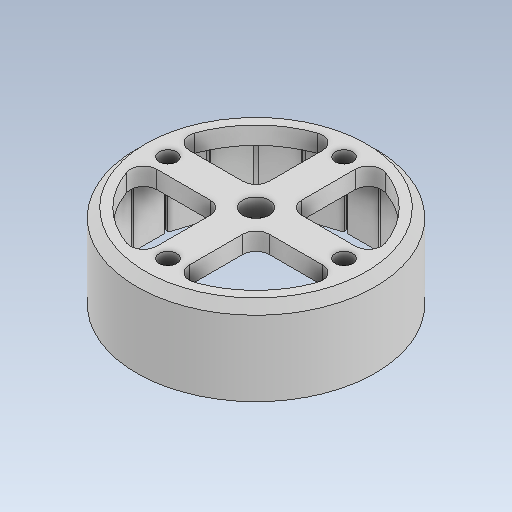
# Autodesk Inventor part: mot_27_1
Saved by Autodesk Inventor 2023 (Build 270158000, 158)
## iProperties
Created: 2020-12-02
Part Number: mot_27_1
Material: Generic
Document SubType Name: Modeling
Designer: Shuang Peng
Density: 1 g/cm^3
Appearance: Default
Author: Shuang Peng
Autodesk Inventor part; units mm, degrees
ref_plane "YZ Plane" through (0, 0, 0) normal (1, 0, 0) x (0, 1, 0)
ref_plane "XZ Plane" through (0, 0, 0) normal (0, 1, 0) x (-1, 0, 0)
ref_plane "XY Plane" through (0, 0, 0) normal (0, 0, 1) x (1, 0, 0)
sketch "Sketch1" plane through (0, 0, 0) normal (0, 1, 0) x (-1, 0, 0)
  circle A0 centre (0, 0) radius 13.55
  dimension "d0" = 27.1
  constraints: 1 centre point, 1 coincident
  measures "d0" diameter of A0
extrude "Extrusion1" add sketch "Sketch1" along normal blind 9.5
sketch "Sketch2" plane through (0, 9.5, 0) normal (0, 1, 0) x (1, 0, 0)
  circle A0 centre (0, 0) radius 13.55 projected
  line L0 (-1.85, -20) -> (1.85, -20)
  line L1 (1.85, -20) -> (1.85, 20)
  line L2 (1.85, 20) -> (-1.85, 20)
  line L3 (-1.85, 20) -> (-1.85, -20)
  line L4 (-1.85, -20) -> (1.85, 20) construction
  line L5 (1.85, -20) -> (-1.85, 20) construction
  line L6 (-20, -1.85) -> (-20, 1.85)
  line L7 (-20, 1.85) -> (20, 1.85)
  line L8 (20, 1.85) -> (20, -1.85)
  line L9 (20, -1.85) -> (-20, -1.85)
  line L10 (-20, -1.85) -> (20, 1.85) construction
  line L11 (-20, 1.85) -> (20, -1.85) construction
  circle A1 centre (0, 0) radius 11.5
  point P0 (1.85, -11.3502)
  point P1 (11.3502, -1.85)
  point P2 (1.85, -1.85)
  point P3 (11.3502, 1.85)
  point P4 (1.85, 11.3502)
  point P5 (1.85, 1.85)
  point P6 (-1.85, 11.3502)
  point P7 (-11.3502, 1.85)
  point P8 (-1.85, 1.85)
  point P9 (-11.3502, -1.85)
  point P10 (-1.85, -11.3502)
  point P11 (-1.85, -1.85)
  dimension "d3" = 3.7
  dimension "d4" = 40
  dimension "d5" = 3.7
  dimension "d6" = 40
  dimension "d7" = 23
  constraints: 24 end point, 4 midpoint, 4 parallel, 3 perpendicular, 1 centre point, 1 coincident, 1 horizontal
  measures "d3" distance of L0.start L0.end
  measures "d4" distance of L1.end L0.end
  measures "d5" distance of L6.start L6.end
  measures "d6" distance of L6.end L7.end
  measures "d7" diameter of A1
extrude "Extrusion2" cut sketch "Sketch2" against normal blind 9.5 contours L7 L1 A1 | A1 L1 L9 | L3 L7 A1 | A1 L9 L3
sketch "Sketch3" plane through (0, 0, 0) normal (0, -1, 0) x (1, 0, 0)
  line L0 (1.85, -11.3502) -> (1.85, -1.85) projected
  line L1 (1.85, -1.85) -> (11.3502, -1.85) projected
  arc A0 (1.85, -11.3502) -> (11.3502, -1.85) centre (0, 0) ccw projected
  line L2 (-11.3502, -1.85) -> (-1.85, -1.85) projected
  line L3 (-1.85, -1.85) -> (-1.85, -11.3502) projected
  arc A1 (-11.3502, -1.85) -> (-1.85, -11.3502) centre (0, 0) ccw projected
  line L4 (1.85, 1.85) -> (1.85, 11.3502) projected
  arc A2 (11.3502, 1.85) -> (1.85, 11.3502) centre (0, 0) ccw projected
  line L5 (11.3502, 1.85) -> (1.85, 1.85) projected
  arc A3 (-1.85, 11.3502) -> (-11.3502, 1.85) centre (0, 0) ccw projected
  line L6 (-1.85, 11.3502) -> (-1.85, 1.85) projected
  line L7 (-1.85, 1.85) -> (-11.3502, 1.85) projected
  circle A4 centre (0, 0) radius 13.55 projected
  circle A5 centre (0, 0) radius 12.7
  circle A6 centre (0, 0) radius 13.55 projected
  dimension "d10" = 0.85
  constraints: 1 centre point, 1 coincident
  measures "d10" radial gap between concentric circles of A6 A5
extrude "Extrusion3" cut sketch "Sketch3" against normal blind 7.5 contours A5
chamfer "Chamfer1" distance 1 angle 45 1 edges at (13.55, 9.5, 0)
sketch "Sketch4" plane through (0, 9.5, 0) normal (0, 1, 0) x (1, 0, 0)
  circle A0 centre (0, 0) radius 1.5
  dimension "d17" = 3
  constraints: 1 centre point, 1 coincident
  measures "d17" diameter of A0
extrude "Extrusion4" cut sketch "Sketch4" against normal blind 7.5
sketch "Sketch5" plane through (0, 7.5, 0) normal (0, -1, 0) x (1, 0, 0)
  circle A0 centre (0, 0) radius 1.5 projected
  circle A1 centre (0, 0) radius 12.7 projected
  line L0 (-11.3502, 1.85) -> (-1.85, 1.85) projected
  arc A2 (-1.85, 11.3502) -> (-11.3502, 1.85) centre (0, 0) ccw projected
  line L1 (-1.85, 1.85) -> (-1.85, 11.3502) projected
  line L2 (1.85, 1.85) -> (11.3502, 1.85) projected
  line L3 (1.85, 11.3502) -> (1.85, 1.85) projected
  arc A3 (11.3502, 1.85) -> (1.85, 11.3502) centre (0, 0) ccw projected
  arc A4 (-11.3502, -1.85) -> (-1.85, -11.3502) centre (0, 0) ccw projected
  line L4 (-1.85, -1.85) -> (-11.3502, -1.85) projected
  line L5 (-1.85, -11.3502) -> (-1.85, -1.85) projected
  line L6 (1.85, -1.85) -> (1.85, -11.3502) projected
  line L7 (11.3502, -1.85) -> (1.85, -1.85) projected
  arc A5 (1.85, -11.3502) -> (11.3502, -1.85) centre (0, 0) ccw projected
  circle A6 centre (0, 0) radius 12.7 projected
  line L8 (0, 0) -> (0, -12.5)
  line L9 (1.75, -12.85) -> (1.75, -12.15)
  line L10 (1.75, -12.15) -> (-1.75, -12.15)
  line L11 (-1.75, -12.15) -> (-1.75, -12.85)
  line L12 (-1.75, -12.85) -> (1.75, -12.85)
  line L13 (1.75, -12.85) -> (-1.75, -12.15) construction
  line L14 (1.75, -12.15) -> (-1.75, -12.85) construction
  dimension "d20" = 12.5
  dimension "d21" = 0.7
  dimension "d22" = 3.5
  constraints: 14 end point, 2 midpoint, 2 parallel, 2 perpendicular, 1 vertical
  measures "d20" distance of L8.start L8.end
  measures "d21" distance of L9.start L9.end
  measures "d22" distance of L10.end L9.end
extrude "Extrusion5" add sketch "Sketch5" along normal blind 7.5 contours L11 L10 L9 A1 | A1 L9 L12 L11 picked at (-0.7783, -12.3288)
pattern_circular "Circular Pattern1" count 20 over 360 about axis through (0, 0, 0) along (0, 1, 0) of "Extrusion5"
sketch "Sketch6" plane through (0, 9.5, 0) normal (0, 1, 0) x (1, 0, 0)
  line L0 (0, 0) -> (0, 10)
  circle A0 centre (0, 10) radius 1
  circle A1 centre (-10, 0) radius 1
  circle A2 centre (0, -10) radius 1
  circle A3 centre (10, 0) radius 1
  dimension "d28" = 10
  dimension "d29" = 2
  dimension "d32" = 360
  constraints: 4 centre point, 2 end point, 1 coincident, 1 vertical, 9 other
  measures "d28" distance of L0.start L0.end
  measures "d29" diameter of A0
extrude "Extrusion6" cut sketch "Sketch6" against normal blind 7.5
fillet "Fillet2" radius 1.5 12 edges at (1.85, 8.5, -1.85) (1.85, 8.5, 1.85) (-1.85, 8.5, -1.85) (-1.85, 8.5, 1.85) (-11.3502, 8.5, 1.85) (11.3502, 8.5, 1.85) (-11.3502, 8.5, -1.85) (11.3502, 8.5, -1.85) (-1.85, 8.5, -11.3502) (-1.85, 8.5, 11.3502) (1.85, 8.5, -11.3502) (1.85, 8.5, 11.3502)
body "Solid1"
